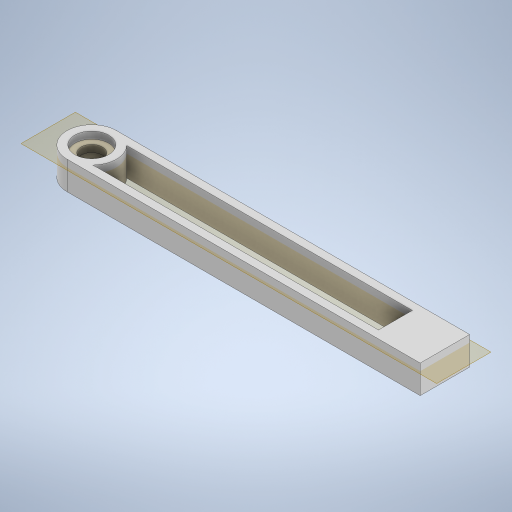
# Autodesk Inventor part: dlon
Saved by Autodesk Inventor 2024.3 (Build 283343000, 343)
## iProperties
Created: 2024-07-21
Part Number: dlon
Material: Ogólny
Document SubType Name: Modeling
Designer: User
Density: 1 g/cm^3
Appearance: Domyślna
Author: User
Autodesk Inventor part; units mm, degrees
ref_plane "YZ Plane" through (0, 0, 0) normal (1, 0, 0) x (0, 1, 0)
ref_plane "XZ Plane" through (0, 0, 0) normal (0, 1, 0) x (-1, 0, 0)
ref_plane "XY Plane" through (0, 0, 0) normal (0, 0, 1) x (1, 0, 0)
sketch "Szkic1" plane through (0, 0, 0) normal (0, 1, 0) x (-1, 0, 0)
  circle A0 centre (0, 0) radius 2.4
  circle A1 centre (0, 0) radius 3.5
  line L0 (0, 3.5) -> (-20, 3.5)
  line L1 (-20, 3.5) -> (-20, -3.5)
  line L2 (-20, -3.5) -> (0, -3.5)
  arc A2 (0, -3.5) -> (0, 3.5) centre (0, 0) ccw
  line L3 (0, 2.4) -> (-6, 2.4)
  line L4 (-6, 2.4) -> (-6, -2.4)
  line L5 (-6, -2.4) -> (0, -2.4)
  line L6 (-6, 2.4) -> (-18, 2.4)
  line L7 (-18, 2.4) -> (-18, -2.4)
  line L8 (-18, -2.4) -> (-6, -2.4)
  line L9 (-6, -2.4) -> (-6, 2.4)
  line L10 (0, 0) -> (-50, 0)
  line L11 (-20, 3.5) -> (-50, 3.5)
  line L12 (-50, 3.5) -> (-50, -3.5)
  line L13 (-50, -3.5) -> (-20, -3.5)
  line L14 (-20, -3.5) -> (-20, 3.5)
  line L15 (-18, 2.4) -> (-43, 2.4)
  line L16 (-43, 2.4) -> (-43, -2.4)
  line L17 (-43, -2.4) -> (-18, -2.4)
  line L18 (-18, -2.4) -> (-18, 2.4)
  point P0 (-2.5475, 2.4)
  point P1 (-2.5475, -2.4)
  dimension "d0" = 4.8
  dimension "d1" = 7
  dimension "d2" = 20
  dimension "d3" = 6
  dimension "d4" = 12
  dimension "d10" = 50
  dimension "d11" = 25
  dimension "d12" = 4.8
  constraints: 38 end point, 7 parallel, 6 point on circle, 6 tangent, 5 horizontal, 5 perpendicular, 3 centre point, 2 coincident
  measures "d0" diameter of A0
  measures "d1" diameter of A1
  measures "d2" distance of L0.start L0.end
  measures "d3" distance of L3.start L3.end
  measures "d4" distance of L8.end L7.end
  measures "d10" distance of L10.start L10.end
  measures "d11" distance of L17.end L16.end
  measures "d12" distance of L16.end L15.end
extrude "Wyciągnięcie proste1" add sketch "Szkic1" along normal blind 4 contours A0 L3 A1 L5 | A0 L10 A1 L3 | L5 A1 L10 A0 | L3 L6 L15 L1 L0 A1 | A1 L2 L1 L17 L8 L5 | L1 L15 L16 L10 L12 L11 | L13 L12 L10 L16 L17 L1
ref_plane "Płaszczyzna konstrukcyjna1" through (0, 3, 0) normal (0, 1, 0) x (1, 0, 0)
sketch "Szkic2" plane through (0, 3, 0) normal (0, 1, 0) x (1, 0, 0)
  circle A0 centre (0, 0) radius 1.5
  circle A1 centre (0, 0) radius 2.4
  dimension "d14" = 3
  constraints: 2 centre point, 2 coincident
  measures "d14" diameter of A0
extrude "Wyciągnięcie proste2" add sketch "Szkic2" against normal blind 1
